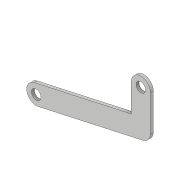
# Autodesk Inventor part: Barra estabilizadora de ascenso
Saved by Autodesk Inventor 2019 (Build 230136000, 136)
## iProperties
Created: 2020-02-06
Part Number: Barra estabilizadora de ascenso
Material: Generic
Document SubType Name: Modeling
Designer: Juan Carlos Botero
Density: 1 g/cm^3
Appearance: Default
Author: Juan Carlos Botero
Autodesk Inventor part; units mm, degrees
ref_plane "YZ Plane" through (0, 0, 0) normal (1, 0, 0) x (0, 1, 0)
ref_plane "XZ Plane" through (0, 0, 0) normal (0, 1, 0) x (-1, 0, 0)
ref_plane "XY Plane" through (0, 0, 0) normal (0, 0, 1) x (1, 0, 0)
sketch "Sketch1" plane through (0, 0, 0) normal (0, 0, 1) x (1, 0, 0)
  circle A0 centre (0, 0) radius 10
  circle A1 centre (-217.9737, -122.4233) radius 10
  line L0 (0, 0) -> (0, -74.3359) construction
  line L1 (-20, 0) -> (-20, -74.3359)
  line L2 (20, -74.3359) -> (20, 0)
  arc A2 (20, 0) -> (-20, 0) centre (0, 0) ccw
  arc A3 (-20, -74.3359) -> (20, -74.3359) centre (0, -74.3359) ccw
  line L3 (0, -74.3359) -> (-217.9737, -122.4233) construction
  line L4 (4.3086, -93.8662) -> (-213.6651, -141.9536)
  line L5 (-222.2823, -102.8929) -> (-4.3086, -54.8055)
  arc A4 (4.3086, -93.8662) -> (-4.3086, -54.8055) centre (0, -74.3359) ccw
  arc A5 (-222.2823, -102.8929) -> (-213.6651, -141.9536) centre (-217.9737, -122.4233) ccw
  point P0 (0, -37.1679)
  point P1 (-108.9869, -98.3796)
  dimension "d1" = 20
  dimension "d6" = 40
  constraints: 16 end point, 8 point on circle, 8 tangent, 6 centre point, 2 equal radius, 2 midpoint, 2 parallel, 1 coincident, 1 vertical
  measures "d1" diameter of A0
  measures "d6" diameter of A3
extrude "Extrusion1" add sketch "Sketch1" along normal blind 6
body "Solid1"
